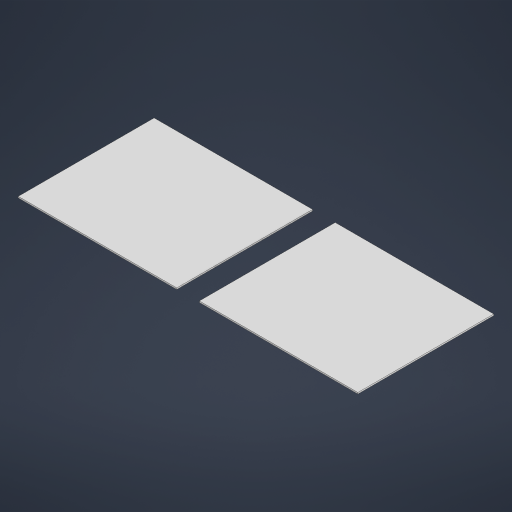
# Autodesk Inventor part: shootingabs
Saved by Autodesk Inventor 2023 (Build 270158000, 158)
## iProperties
Created: 2023-02-25
Part Number: shootingabs
Material: Generic
Document SubType Name: Modeling
Designer: Windows Macbook
Density: 1 g/cm^3
Appearance: Default
Author: Windows Macbook
Autodesk Inventor part; units mm, degrees
ref_plane "YZ Plane" through (0, 0, 0) normal (1, 0, 0) x (0, 1, 0)
ref_plane "XZ Plane" through (0, 0, 0) normal (0, 1, 0) x (-1, 0, 0)
ref_plane "XY Plane" through (0, 0, 0) normal (0, 0, 1) x (1, 0, 0)
sketch "Sketch1" plane through (0, 0, 0) normal (0, 1, 0) x (-1, 0, 0)
  line L0 (0, 0) -> (0, -152.4)
  line L1 (0, -152.4) -> (177.8, -152.4)
  line L2 (177.8, -152.4) -> (177.8, 0)
  line L3 (177.8, 0) -> (0, 0)
  line L4 (203.2, 0) -> (203.2, -152.4)
  line L5 (203.2, -152.4) -> (381, -152.4)
  line L6 (381, -152.4) -> (381, 0)
  line L7 (381, 0) -> (203.2, 0)
  dimension "d0" = 152.4
  dimension "d1" = 177.8
  dimension "d2" = 25.4
  dimension "d3" = 177.8
  constraints: 16 end point, 6 perpendicular, 1 vertical
  measures "d0" distance of L0.start L0.end
  measures "d1" distance of L0.end L1.end
  measures "d2" distance of L2.end L4.start
  measures "d3" distance of L4.end L5.end
extrude "Extrusion1" add sketch "Sketch1" along normal blind 1.5875
body "Solid1"
